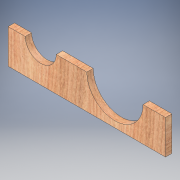
# Autodesk Inventor part: cannon support front
Saved by Autodesk Inventor 2018 (Build 220112000, 112)
## iProperties
Created: 2017-05-03
Part Number: cannon support front
Material: Generic
Document SubType Name: Modeling
Designer: gsegs
Density: 1 g/cm^3
Appearance: Birch - Natural Polished
Author: gsegs
Autodesk Inventor part; units mm, degrees
ref_plane "YZ Plane" through (0, 0, 0) normal (1, 0, 0) x (0, 1, 0)
ref_plane "XZ Plane" through (0, 0, 0) normal (0, 1, 0) x (-1, 0, 0)
ref_plane "XY Plane" through (0, 0, 0) normal (0, 0, 1) x (1, 0, 0)
sketch "Sketch1" plane through (0, 0, 0) normal (0, 0, 1) x (1, 0, 0)
  line L0 (0, 101.6) -> (50.8, 101.6)
  line L1 (466.725, 101.6) -> (466.725, 0)
  line L2 (466.725, 0) -> (0, 0)
  line L3 (0, 0) -> (0, 101.6)
  arc A0 (50.8, 101.6) -> (142.875, 101.6) centre (96.8375, 101.6) ccw
  arc A1 (233.3625, 101.6) -> (400.05, 101.6) centre (316.7062, 101.6) ccw
  line L4 (50.8, 101.6) -> (142.875, 101.6) construction
  line L5 (142.875, 101.6) -> (233.3625, 101.6)
  line L6 (233.3625, 101.6) -> (400.05, 101.6) construction
  line L7 (400.05, 101.6) -> (466.725, 101.6)
  dimension "d0" = 466.725
  dimension "d1" = 101.6
  dimension "d2" = 50.8
  dimension "d3" = 90.4875
  dimension "d4" = 66.675
  dimension "d5" = 92.075
  dimension "d6" = 166.6875
  constraints: 16 end point, 10 point on line, 6 parallel, 5 horizontal, 5 perpendicular, 4 point on circle, 2 centre point, 2 midpoint, 1 coincident
  measures "d0" distance between parallel lines of L1 L3
  measures "d1" distance between parallel lines of L2 L0
  measures "d2" distance of L0.end L0.start
  measures "d3" distance of L5.end L4.end
  measures "d4" distance of L1.start L6.end
  measures "d5" distance of L4.end L0.end
  measures "d6" distance of L6.end L5.end
extrude "Extrusion1" add sketch "Sketch1" along normal blind 19.05
body "Solid1"
